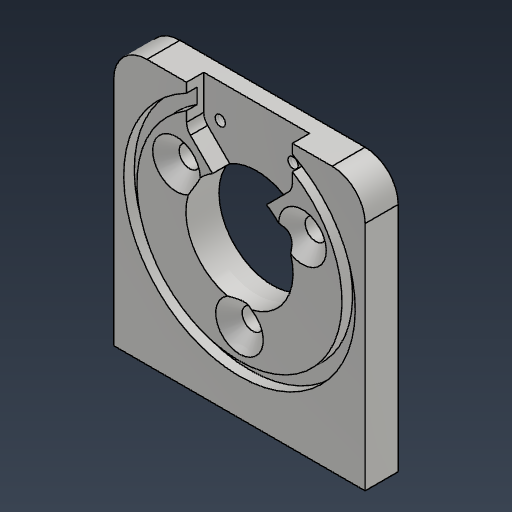
# Autodesk Inventor part: Lagerbock
Saved by Autodesk Inventor 2023.1 (Build 271208000, 208)
## iProperties
Part Number: Lagerbock
Material: Aluminium 6061
Document SubType Name: Modeling
Designer: rYan
Density: 2.7 g/cm^3
Appearance: Aluminium - flach
Mass: 15.0828 g
Surface Area: 41.0098 cm^2
Volume: 5.5862 cm^3
Author: rYan
Autodesk Inventor part; units mm, degrees
ref_plane "YZ Plane" through (0, 0, 0) normal (1, 0, 0) x (0, 1, 0)
ref_plane "XZ Plane" through (0, 0, 0) normal (0, 1, 0) x (-1, 0, 0)
ref_plane "XY Plane" through (0, 0, 0) normal (0, 0, 1) x (1, 0, 0)
sketch "Skizze1" plane through (0, 0, 0) normal (0, 1, 0) x (-1, 0, 0)
  line L0 (6, 0) -> (-32, 0)
  line L1 (-32, 0) -> (-32, 40)
  line L2 (-32, 40) -> (6, 40)
  line L3 (6, 40) -> (6, 0)
  line L4 (0, -18.996) -> (0, 55.666) projected
  circle A0 centre (-13, 23) radius 0.5
  circle A1 centre (-13, 23) radius 22 construction
  line L5 (0, -8.33) -> (0, 0) construction
  line L6 (-13, 23) -> (-13, 1) construction
  line L7 (9, 23) -> (-35, 23) construction
  dimension "d0" = 40
  dimension "d1" = 38
  dimension "d83" = 1
  dimension "d85" = 44
  dimension "d138" = 13
  dimension "d140" = 8.33
  dimension "d176" = 23
  constraints: 14 end point, 3 point on circle, 2 centre point, 2 horizontal, 2 parallel, 2 perpendicular, 2 point on line, 1 coincident, 1 midpoint, 1 vertical, 1 other
  measures "d0" distance of L2.end L0.start
  measures "d1" distance of L1.end L2.end
  measures "d83" diameter of A0
  measures "d85" diameter of A1
  measures "d138" distance between parallel lines of L6 L4
  measures "d140" distance from line of L5.start L0
  measures "d176" distance between parallel lines of L0 L7
extrude "Extrusion1" add sketch "Skizze1" along normal mid plane 5
sketch "Skizze12" plane through (0, -2.5, 0) normal (0, -1, 0) x (1, 0, 0)
  circle A0 centre (13, 23) radius 0.5 projected
  circle A1 centre (13, 23) radius 0.5 projected
  point P0 (0, 0)
  constraints: 1 coincident
hole "Motormitte" at (13, -2.5, 23) direction (0, 1, 0) diameter 16.2 end through all
sketch "Skizze13" plane through (0, -2.5, 0) normal (0, -1, 0) x (1, 0, 0)
  circle A0 centre (13, 23) radius 0.5 projected
  circle A1 centre (13, 23) radius 0.5 construction
  circle A2 centre (13, 23) radius 11 construction
  line L0 (13, 23) -> (13, 12) construction
  point P0 (0, 0)
  dimension "d106" = 22
  constraints: 2 coincident, 2 end point, 1 vertical, 1 vertical alignment, 2 other
hole "Motorschraube" at (13, -2.5, 12) direction (0, 1, 0) diameter 3.2 end through all countersink diameter 7.2 countersink angle 90
pattern_circular "Motorschrauben" count 3 over 360 about axis through (13, 0, 23) along (0, 1, 0) of "Motorschraube"
sketch "Skizze14" plane through (32, 2.5, 0) normal (0, 0, -1) x (-1, 0, 0)
  line L0 (32, -6) -> (32, 1) projected
  line L1 (24.9263, -5) -> (13.0737, -5) projected
  line L2 (27.1, 0) -> (27.1, 0) projected
  line L3 (19, -5) -> (19, 0) construction
  line L4 (31, -2.5) -> (7, -2.5) construction
  line L5 (22.6, -5) -> (15.4, -5) projected
  line L6 (38, 0) -> (38, -5) projected
  line L7 (0, 0) -> (38, 0) projected
  line L8 (0, 0) -> (0, -5) projected
  line L9 (38, -5) -> (0, -5) projected
  point P0 (32, -2.5)
  point P1 (19, -2.5)
  point P2 (17.1813, -5)
  point P3 (20.8187, -5)
  point P4 (19, -2.5)
  dimension "d139" = 24
  constraints: 4 end point, 4 midpoint, 1 coincident, 1 horizontal
  measures "d139" distance of L4.start L4.end
hole "Montage" at (1, 0, 0) at (25, 0, 0) at (13, 0, 0) direction (0, 0, 1) diameter 2.459 depth 5.2 tip angle 118 thread size "M3x0.5" class "6H" standard "ISO Metric profile"
fillet "Rundung1" radius 5 2 edges at (32, 0, 40) (-6, 0, 40)
sketch "Skizze21" plane through (0, -2.5, 0) normal (0, -1, 0) x (1, 0, 0)
  arc A0 (5.255, 25.3715) -> (11.1813, 15.1068) centre (13, 23) ccw projected
  circle A1 centre (13, 23) radius 15.5
  circle A2 centre (13, 23) radius 17.5
  point P0 (0, 0)
  dimension "d177" = 31
  dimension "d178" = 35
  constraints: 2 centre point, 2 coincident
  measures "d177" diameter of A1
  measures "d178" diameter of A2
extrude "Extrusion8" cut sketch "Skizze21" against normal blind 1.6
sketch "Skizze22" plane through (13, -2.5, 23) normal (0, -1, 0) x (1, 0, 0)
  circle A0 centre (-5.5, 11.9245) radius 2 construction
  circle A1 centre (5.5, 11.9245) radius 2 construction
  line L0 (-2.0788, 13.9499) -> (1.9212, 13.9499) construction
  line L1 (1.9212, 13.9499) -> (1.9212, 8.7499) construction
  line L2 (1.9212, 8.7499) -> (-2.0788, 8.7499) construction
  line L3 (-2.0788, 8.7499) -> (-2.0788, 13.9499) construction
  line L4 (-8, 10.9245) -> (-4.0755, 7)
  line L5 (-4.0755, 7) -> (4.0755, 7)
  line L6 (4.0755, 7) -> (8, 10.9245)
  line L7 (8, 10.9245) -> (8, 17)
  line L8 (8, 17) -> (-8, 17)
  line L9 (-8, 17) -> (-8, 10.9245)
  arc A2 (1.8187, -7.8932) -> (7.745, 2.3715) centre (0, 0) ccw construction
  line L10 (0, 0) -> (0, 17) construction
  line L11 (-14, 17) -> (14, 17) construction
  circle A3 centre (0, 0) radius 12.7 construction
  line L12 (-2.0788, 11.3499) -> (1.9212, 11.3499) construction
  circle A4 centre (0, 0) radius 10.2 construction
  arc A5 (5.9263, 5.5216) -> (-5.9263, 5.5216) centre (0, 0) ccw construction
  line L13 (-8, 10.9245) -> (8, 10.9245) construction
  point P0 (-13, -23)
  dimension "d181" = 4
  dimension "d182" = 4
  dimension "d183" = 5.2
  dimension "d184" = 4
  dimension "d185" = 25.4
  dimension "d186" = 20.4
  dimension "d187" = 45
  dimension "d188" = 7
  dimension "d189" = 16
  dimension "d192" = 11
  dimension "d193" = 1
  constraints: 27 end point, 4 centre point, 3 horizontal, 3 midpoint, 3 perpendicular, 2 coincident, 2 parallel, 1 collinear, 1 point on circle, 1 symmetric about line, 2 other
  measures "d181" diameter of A0
  measures "d182" diameter of A1
  measures "d183" distance of L0.end L1.end
  measures "d184" distance of L0.start L0.end
  measures "d185" diameter of A3
  measures "d186" diameter of A4
  measures "d187" angle of L4 L5
  measures "d188" distance from line of A3.centre L5
  measures "d189" distance of L7.end L8.end
  measures "d192" distance of A1.centre A0.centre
  measures "d193" distance from line of L13 A1.centre
extrude "Extrusion9" cut sketch "Skizze22" against normal blind 2.6
sketch "Skizze23" plane through (13, 0.1, 23) normal (0, -1, 0) x (1, 0, 0)
  arc A0 (4.0755, 7) -> (-4.0755, 7) centre (0, 0) ccw projected
  line L0 (8, 10.9245) -> (4.0755, 7) projected
  line L1 (8, 17) -> (8, 10.9245) projected
  line L2 (-8, 17) -> (8, 17) projected
  line L3 (-8, 10.9245) -> (-8, 17) projected
  line L4 (-4.0755, 7) -> (-8, 10.9245) projected
  line L5 (-8, 10.9245) -> (-8, 17) construction
  line L6 (-8, 10.9245) -> (8, 10.9245) construction
  line L7 (0, 0) -> (0, 17) construction
  line L8 (-14, 17) -> (14, 17) construction
  point P0 (-13, -23)
  point P1 (-5.5, 11.9245)
  point P2 (5.5, 11.9245)
  dimension "d194" = 11
  dimension "d195" = 1
  constraints: 4 end point, 1 midpoint, 1 perpendicular, 1 symmetric about line
  measures "d194" distance of point (5.5, 11.924) point (-5.5, 11.924)
  measures "d195" distance from line of L6 point (5.5, 11.924)
hole "Bohrung13" at (7.5, 0.1, 34.9245) at (18.5, 0.1, 34.9245) direction (0, 1, 0) diameter 1.567 end through all thread size "M2x0.4" class "6H" standard "ISO Metric profile"
fillet "Rundung2" radius 2 2 edges at (5, -1.2, 33.9245) (21, -1.2, 33.9245)
